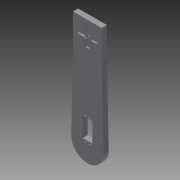
# Autodesk Inventor part: FrontUpperLeg
Saved by Autodesk Inventor 2014 SP1 (Build 180222100, 222)
## iProperties
Created: 2013-09-20
Part Number: FrontUpperLeg
Material: Generic
Document SubType Name: Modeling
Designer: Medrimonia
Density: 1 g/cm^3
Appearance: Default
Author: Medrimonia
Autodesk Inventor part; units mm, degrees
ref_plane "YZ Plane" through (0, 0, 0) normal (1, 0, 0) x (0, 1, 0)
ref_plane "XZ Plane" through (0, 0, 0) normal (0, 1, 0) x (-1, 0, 0)
ref_plane "XY Plane" through (0, 0, 0) normal (0, 0, 1) x (1, 0, 0)
sketch "Sketch1" plane through (0, 0, 0) normal (0, 1, 0) x (-1, 0, 0)
  line L0 (-17.75, -17.75) -> (17.75, -17.75)
  line L1 (17.75, -17.75) -> (17.75, 17.75)
  line L2 (17.75, 17.75) -> (-17.75, 17.75)
  line L3 (-17.75, 17.75) -> (-17.75, -17.75)
  line L4 (-17.75, -17.75) -> (17.75, 17.75) construction
  line L5 (17.75, -17.75) -> (-17.75, 17.75) construction
  line L6 (-2.45, -12.65) -> (2.45, -12.65) construction
  line L7 (2.45, -12.65) -> (2.45, 12.65) construction
  line L8 (2.45, 12.65) -> (-2.45, 12.65) construction
  line L9 (-2.45, 12.65) -> (-2.45, -12.65) construction
  line L10 (-2.45, -12.65) -> (2.45, 12.65) construction
  line L11 (2.45, -12.65) -> (-2.45, 12.65) construction
  line L12 (-12.65, -2.45) -> (12.65, -2.45) construction
  line L13 (12.65, -2.45) -> (12.65, 2.45) construction
  line L14 (12.65, 2.45) -> (-12.65, 2.45) construction
  line L15 (-12.65, 2.45) -> (-12.65, -2.45) construction
  line L16 (-12.65, -2.45) -> (12.65, 2.45) construction
  line L17 (12.65, -2.45) -> (-12.65, 2.45) construction
  line L18 (-12.85, -2.65) -> (12.85, -2.65)
  line L19 (12.85, -2.65) -> (12.85, 2.65)
  line L20 (12.85, 2.65) -> (-12.85, 2.65)
  line L21 (-12.85, 2.65) -> (-12.85, -2.65)
  line L22 (-12.85, -2.65) -> (12.85, 2.65) construction
  line L23 (12.85, -2.65) -> (-12.85, 2.65) construction
  line L24 (-2.65, -12.85) -> (2.65, -12.85)
  line L25 (2.65, -12.85) -> (2.65, 12.85)
  line L26 (2.65, 12.85) -> (-2.65, 12.85)
  line L27 (-2.65, 12.85) -> (-2.65, -12.85)
  line L28 (-2.65, -12.85) -> (2.65, 12.85) construction
  line L29 (2.65, -12.85) -> (-2.65, 12.85) construction
  point P0 (0, 0)
  point P1 (0, 0)
  dimension "d0" = 35.5
  dimension "d1" = 4.9
  dimension "d2" = 10.2
  dimension "d3" = 0.2
  dimension "d4" = 0.2
  constraints: 60 end point, 12 midpoint, 10 parallel, 10 perpendicular, 5 horizontal
  measures "d0" distance of L1.end L2.end
  measures "d1" distance of L14.end L12.start
  measures "d2" distance between parallel lines of L13 L7
  measures "d3" distance between parallel lines of L25 L7
  measures "d4" distance between parallel lines of L26 L8
extrude "Extrusion1" add sketch "Sketch1" along normal blind 1.9
sketch "Sketch2" plane through (0, 1.9, 0) normal (0, 1, 0) x (1, 0, 0)
  line L0 (17.75, 17.75) -> (-17.75, 17.75) projected
  line L1 (-17.75, 17.75) -> (-17.75, -17.75) projected
  line L2 (-17.75, -17.75) -> (17.75, -17.75) projected
  line L3 (17.75, -17.75) -> (17.75, 17.75) projected
  circle A0 centre (0, 0) radius 1.5
  dimension "d7" = 3
  constraints: 1 centre point, 1 coincident
  measures "d7" diameter of A0
extrude "Extrusion2" add sketch "Sketch2" along normal blind 2
sketch "Sketch3" plane through (0, 3.9, 0) normal (0, 1, 0) x (1, 0, 0)
  circle A0 centre (0, 0) radius 1.5 projected
  line L0 (17.75, 17.75) -> (-17.75, 17.75) projected
  line L1 (-17.75, 17.75) -> (-17.75, -17.75) projected
  line L2 (-17.75, -17.75) -> (17.75, -17.75) projected
  line L3 (17.75, -17.75) -> (17.75, 17.75) projected
  circle A1 centre (0, 0) radius 2.75
  dimension "d10" = 5.5
  constraints: 1 centre point, 1 coincident
  measures "d10" diameter of A1
extrude "Extrusion3" add sketch "Sketch3" along normal blind 2.5 contours L3 L2 L1 L0
chamfer "Chamfer1" distance 2 angle 45 1 edges at (-2.65, 0.95, -2.65)
fillet "Fillet1" radius 2.45 1 edges at (-12.85, 0.95, -2.65)
fillet "Fillet2" radius 2.45 1 edges at (-2.65, 0.95, -12.85)
chamfer "Chamfer2" distance 2 angle 45 1 edges at (2.65, 0.95, -2.65)
chamfer "Chamfer3" distance 2 angle 45 1 edges at (2.65, 0.95, 2.65)
fillet "Fillet3" radius 2.45 1 edges at (12.85, 0.95, -2.65)
fillet "Fillet4" radius 2.45 1 edges at (2.65, 0.95, -12.85)
fillet "Fillet5" radius 2.45 1 edges at (12.85, 0.95, 2.65)
fillet "Fillet6" radius 2.45 1 edges at (2.65, 0.95, 12.85)
chamfer "Chamfer4" distance 2 angle 45 1 edges at (-2.65, 0.95, 2.65)
fillet "Fillet7" radius 2.45 2 edges at (-2.65, 0.95, 12.85) (-12.85, 0.95, 2.65)
sketch "Sketch4" plane through (0, 0, 0) normal (0, -1, 0) x (1, 0, 0)
  line L0 (17.75, -17.75) -> (-17.75, -17.75) projected
  line L1 (-10.4, 2.65) -> (-4.65, 2.65) projected
  line L2 (-17.75, -17.75) -> (-20, -116.15)
  line L3 (-20, -116.15) -> (20, -116.15)
  line L4 (20, -116.15) -> (17.75, -17.75)
  line L5 (0, 0) -> (0, -92.3376) construction
  arc A0 (-20, -116.15) -> (20, -116.15) centre (0, -116.15) ccw
  dimension "d32" = 116.15
  dimension "d33" = 40
  constraints: 8 end point, 2 point on circle, 1 centre point, 1 midpoint, 1 parallel, 1 perpendicular, 1 other
  measures "d32" distance from line of L3 L5.start
  measures "d33" distance of L2.end L3.end
extrude "Extrusion4" add sketch "Sketch4" against normal up to surface (6.4 mm away)
sketch "Sketch5" plane through (0, 0, 0) normal (0, -1, 0) x (1, 0, 0)
  line L0 (-5.7, -88.25) -> (5.7, -88.25) construction
  line L1 (5.7, -88.25) -> (5.7, -111.75) construction
  line L2 (5.7, -111.75) -> (-5.7, -111.75) construction
  line L3 (-5.7, -111.75) -> (-5.7, -88.25) construction
  line L4 (0, 0) -> (0, -72.1654) construction
  line L5 (-5.7, -88.25) -> (-5.7, -83.85) construction
  line L6 (-5.7, -83.85) -> (5.7, -83.85) construction
  line L7 (5.7, -83.85) -> (5.7, -88.25) construction
  line L8 (5.7, -111.75) -> (5.7, -116.15) construction
  line L9 (5.7, -116.15) -> (-5.7, -116.15) construction
  line L10 (-5.7, -116.15) -> (-5.7, -111.75) construction
  circle A0 centre (-2.7, -85.85) radius 1.3
  circle A1 centre (2.7, -85.85) radius 1.3
  line L11 (-17.4512, -100) -> (18.2205, -100) construction
  circle A2 centre (-2.7, -114.15) radius 1.3
  circle A3 centre (2.7, -114.15) radius 1.3
  line L12 (-5.9, -88.05) -> (5.9, -88.05)
  line L13 (5.9, -88.05) -> (5.9, -111.95)
  line L14 (5.9, -111.95) -> (-5.9, -111.95)
  line L15 (-5.9, -111.95) -> (-5.9, -88.05)
  dimension "d36" = 11.4
  dimension "d37" = 23.5
  dimension "d38" = 3
  dimension "d39" = 2.4
  dimension "d40" = 4.4
  dimension "d41" = 0.2
  dimension "d42" = 0.2
  dimension "d43" = 100
  dimension "d44" = 2.6
  constraints: 32 end point, 8 parallel, 5 perpendicular, 4 centre point, 3 symmetric about line, 2 horizontal, 1 collinear, 8 other
  measures "d36" distance between parallel lines of L1 L3
  measures "d37" distance between parallel lines of L2 L0
  measures "d38" distance from line of L5 A0.centre
  measures "d39" distance from line of A3.centre L2
  measures "d40" distance between parallel lines of L0 L6
  measures "d41" distance between parallel lines of L0 L12
  measures "d42" distance between parallel lines of L1 L13
  measures "d43" distance from line of L11 L4.start
  measures "d44" diameter of A1
extrude "Extrusion5" cut sketch "Sketch5" against normal through all
equation "\"d0\" = 3 * ServoArmLength + ServoArmWidth"
equation "\"d1\" = ServoArmWidth"
equation "\"d2\" = ServoArmLength"
equation "\"d3\" = ServoArmSpacing"
equation "\"d4\" = ServoArmSpacing"
equation "\"d5\" = ServoArmThickness"
equation "\"d7\" = ServoArmHoleRequired"
equation "\"d8\" = MinimalThickness"
equation "\"d10\" = ServoArmHeadScrewTrace"
equation "\"d11\" = ServoArmHeadScrewThickness"
equation "\"d13\" = ServoArmInternFillet"
equation "\"d16\" = ServoArmExternFillet"
equation "\"d17\" = ServoArmExternFillet"
equation "\"d18\" = ServoArmInternFillet"
equation "\"d21\" = ServoArmInternFillet"
equation "\"d24\" = ServoArmExternFillet"
equation "\"d25\" = ServoArmExternFillet"
equation "\"d26\" = ServoArmExternFillet"
equation "\"d27\" = ServoArmExternFillet"
equation "\"d28\" = ServoArmInternFillet"
equation "\"d31\" = ServoArmExternFillet"
equation "\"d32\" = 0.5 * ServoCoreLength + FrontUpperLegLength + ServoFixationLength"
equation "\"d33\" = FrontUpperLegKneeWidth"
equation "\"d36\" = ServoCoreWidth"
equation "\"d37\" = ServoCoreLength"
equation "\"d38\" = ServoEdgeToFixation"
equation "\"d39\" = ServoCoreToFixation"
equation "\"d40\" = ServoFixationLength"
equation "\"d41\" = ServoTraceSpacing"
equation "\"d42\" = ServoTraceSpacing"
equation "\"d43\" = FrontUpperLegLength"
equation "\"d44\" = ServoScrewDiameterRequired"
equation "\"FrontUpperLegLength\" = 100"
equation "\"FrontUpperLegKneeWidth\" = 40"
equation "\"ServoTraceSpacing\" = 0.2"
equation "\"ServoArmLength\" = 10.2"
equation "\"ServoArmWidth\" = 4.9"
equation "\"ServoArmSpacing\" = 0.2"
equation "\"ServoArmThickness\" = 1.9"
equation "\"ServoArmHoleRequired\" = 3"
equation "\"MinimalThickness\" = 2"
equation "\"ServoArmHeadScrewTrace\" = 5.5"
equation "\"ServoArmHeadScrewThickness\" = 2.5"
equation "\"ServoArmInternFillet\" = 2"
equation "\"ServoArmExternFillet\" = 2.45"
equation "\"ServoCoreLength\" = 23.5"
equation "\"ServoFixationLength\" = 4.4"
equation "\"ServoCoreWidth\" = 11.4"
equation "\"ServoEdgeToFixation\" = 3"
equation "\"ServoCoreToFixation\" = 2.4"
equation "\"ServoScrewDiameterRequired\" = 2.6"
body "Solid1"
